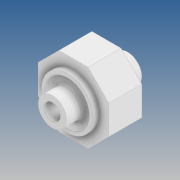
# Autodesk Inventor part: 2112_Adjustment Nut_V1
Saved by Autodesk Inventor 2020 (Build 240168000, 168)
## iProperties
Created: 2019-11-08
Part Number: 2112_Adjustment Nut_V1
Material: ABS Plastic
Document SubType Name: Modeling
Designer: RFLab
Density: 1.06 g/cm^3
Appearance: Smooth - White
Author: RFLab
Autodesk Inventor part; units mm, degrees
ref_plane "YZ Plane" through (0, 0, 0) normal (1, 0, 0) x (0, 1, 0)
ref_plane "XZ Plane" through (0, 0, 0) normal (0, 1, 0) x (-1, 0, 0)
ref_plane "XY Plane" through (0, 0, 0) normal (0, 0, 1) x (1, 0, 0)
sketch "Sketch1" plane through (0, 0, 0) normal (0, 0, 1) x (1, 0, 0)
  circle A0 centre (0, 0) radius 11
  dimension "d0" = 22
  constraints: 1 centre point, 1 coincident
  measures "d0" diameter of A0
extrude "Extrusion1" add sketch "Sketch1" along normal blind 3
sketch "Sketch2" plane through (0, 0, 0) normal (0, 0, -1) x (-1, 0, 0)
  circle A0 centre (0, 0) radius 3.4
  dimension "d3" = 6.8
  constraints: 1 centre point, 1 coincident
  measures "d3" diameter of A0
extrude "Extrusion2" cut sketch "Sketch2" against normal through all
sketch "Sketch3" plane through (0, 0, 3) normal (0, 0, 1) x (1, 0, 0)
  circle A0 centre (0, 0) radius 3.4 projected
  circle A1 centre (0, 0) radius 6
  dimension "d6" = 12
  constraints: 1 centre point, 1 coincident
  measures "d6" diameter of A1
extrude "Extrusion3" add sketch "Sketch3" along normal blind 6
sketch "Sketch4" plane through (0, 0, 3) normal (0, 0, 1) x (1, 0, 0)
  circle A0 centre (0, 0) radius 9.375
  circle A1 centre (0, 0) radius 11
  dimension "d9" = 18.75
  dimension "d13" = 22
  constraints: 2 centre point, 2 coincident
  measures "d9" diameter of A0
  measures "d13" diameter of A1
extrude "Extrusion4" add sketch "Sketch4" along normal blind 0.5
sketch "Sketch5" plane through (0, 0, 0) normal (1, 0, 0) x (0, 1, 0)
  line L0 (-6, 3) -> (6, 3) projected
  line L1 (9.375, 3) -> (-9.375, 3) projected
  line L2 (-6, 3) -> (-9.375, 3)
  arc A0 (-9.375, 3) -> (-6, 3) centre (-7.6875, 3) ccw
  line L3 (0, -0.6) -> (0, 3.6) projected
  point P0 (0, 0)
  constraints: 2 end point, 2 point on circle, 1 centre point, 1 horizontal, 1 midpoint
revolve "Revolution1" cut sketch "Sketch5" angle 360 about axis through (0, 0, -10) along (0, 0, 1)
sketch "Sketch6" plane through (0, 0, 0) normal (0, 0, -1) x (-1, 0, 0)
  line L0 (-15, -15) -> (15, -15)
  line L1 (15, -15) -> (15, 15)
  line L2 (15, 15) -> (-15, 15)
  line L3 (-15, 15) -> (-15, -15)
  point P0 (0, 0)
  dimension "d14" = 30
  dimension "d15" = 30
  dimension "d16" = 15
  dimension "d17" = 15
  constraints: 8 end point, 2 parallel, 1 horizontal, 1 perpendicular
  measures "d14" distance of L1.end L2.end
  measures "d15" distance of L2.end L0.start
  measures "d16" distance from line of L3 point (0, 0)
  measures "d17" distance from line of L2 point (0, 0)
extrude "Extrusion5" add sketch "Sketch6" along normal blind 7
mirror "Mirror1" about plane through (0, 0, -7) normal (0, 0, -1) of "Extrusion5", "Extrusion1", "Extrusion3", "Extrusion2", "Extrusion4", "Revolution1"
sketch "Sketch8" plane through (0, 0, 3.5) normal (0, 0, 1) x (1, 0, 0)
  circle A0 centre (0, 0) radius 11.0166
  circle A1 centre (0, 0) radius 9.394
  circle A2 centre (0, 0) radius 6 projected
  circle A3 centre (0, 0) radius 9.286
  constraints: 3 centre point, 3 coincident
extrude "Extrusion7" cut sketch "Sketch8" against normal blind 0.9 contours A0 | A1
chamfer "Chamfer1" distance 8.8 angle 45 4 edges at (15, 15, -7) (15, -15, -7) (-15, -15, -7) (-15, 15, -7)
sketch "Sketch7" plane through (0, 0, 0) normal (0, 0, 1) x (1, 0, 0)
  circle A0 centre (0, 0) radius 3.4 projected
  circle A1 centre (0, 0) radius 2.395
  constraints: 1 centre point, 1 coincident
extrude "Extrusion6" cut sketch "Sketch7" against normal through all contours A0 | A1
sketch "Sketch9" plane through (0, 0, -17.5) normal (0, 0, -1) x (-1, 0, 0)
  circle A0 centre (0, 0) radius 9.2674
  circle A1 centre (0, 0) radius 11.0048
  constraints: 2 centre point, 2 coincident
extrude "Extrusion8" cut sketch "Sketch9" against normal blind 0.9
sketch "Sketch10" plane through (0, 0, -16.6) normal (0, 0, -1) x (-1, 0, 0)
  circle A0 centre (0, 0) radius 3.4
  circle A1 centre (0, 0) radius 2.8
  dimension "d29" = 5.6
  dimension "d30" = 6.8
  constraints: 2 centre point, 2 coincident
  measures "d29" diameter of A1
  measures "d30" diameter of A0
extrude "Extrusion9" add sketch "Sketch10" against normal blind 19.2
fillet "Fillet1" radius 0.3 3 edges at (0, 3.4, -16.6) (0, -3.4, -16.6) (2.8, 0, -16.6)
fillet "Fillet2" radius 0.3 2 edges at (3.4, 0, 2.6) (2.8, 0, 2.6)
equation "\"d16\" = 0.5 * d14"
equation "\"d17\" = 0.5 * d15"
body "Solid1"
